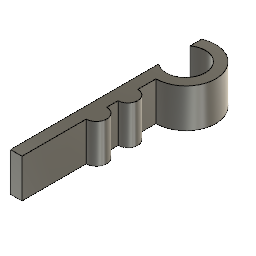
eth_cable_support (Autodesk Fusion 360 design; units mm, degrees)
Autodesk Fusion 360 part; units mm, degrees
sketch "Sketch1" plane through (0, 0, 0) normal (0, 0, 1) x (1, 0, 0)
  line L0 (-3.5, 40) -> (-5, 40)
  arc A0 (-3.5, 57.2195) -> (-5, 64.5984) centre (-3.5, 61.0614) ccw
  arc A1 (-5, 59.0614) -> (-5, 63.0614) centre (-3.5, 61.0614) ccw
  line L1 (-5, 40) -> (-5, 59.0614)
  line L2 (-5, 63.0614) -> (-5, 64.5984)
  line L3 (-3.5, 65) -> (-3.5, 64.9033)
  arc A2 (-3.5, 52.3582) -> (-3.5, 54.8851) centre (-3.5, 53.6216) ccw
  line L4 (-3.5, 57.2195) -> (-3.5, 54.8851)
  line L5 (-3.5, 52.3582) -> (-3.5, 50.9004)
  line L6 (-3.5, 48.2617) -> (-3.5, 40)
  arc A3 (-3.5, 48.2617) -> (-3.5, 50.9004) centre (-3.5, 49.5811) ccw
  dimension "d3" = 5
  constraint vertical L3
  constraint horizontal L0
  constraint vertical L1
  constraint coincident A0.centre L3
  constraint concentric A0 A1
  constraint coincident A0.end L1
  constraint coincident A1.end L1
  constraint collinear L1 L2
  constraint collinear L3 L4
  constraint coincident A0 L3.end
  constraint coincident A3.centre L4
  constraint coincident A2.centre L4
  constraint coincident A2.start L4
  constraint collinear L4 L5
  constraint collinear L5 L6
  measures "d3" diameter of A1
extrude "Extrude1" add sketch "Sketch1" along normal blind 5
